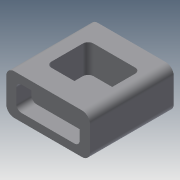
# Autodesk Inventor part: Part1
Saved by Autodesk Inventor 2015 (Build 190159000, 159)
## iProperties
Created: 2016-11-01
Part Number: Part1
Material: Generic
Document SubType Name: Modeling
Designer: Aniket Pant
Density: 1 g/cm^3
Appearance: Default
Author: Aniket Pant
Autodesk Inventor part; units mm, degrees
ref_plane "YZ Plane" through (0, 0, 0) normal (1, 0, 0) x (0, 1, 0)
ref_plane "XZ Plane" through (0, 0, 0) normal (0, 1, 0) x (-1, 0, 0)
ref_plane "XY Plane" through (0, 0, 0) normal (0, 0, 1) x (1, 0, 0)
sketch "Sketch1" plane through (0, 0, 0) normal (0, 0, 1) x (1, 0, 0)
  line L0 (7.62, 0) -> (72.898, 0)
  line L1 (80.518, 7.62) -> (80.518, 31.242)
  line L2 (72.898, 38.862) -> (7.62, 38.862)
  line L3 (0, 31.242) -> (0, 7.62)
  arc A0 (7.62, 38.862) -> (0, 31.242) centre (7.62, 31.242) ccw
  arc A1 (80.518, 31.242) -> (72.898, 38.862) centre (72.898, 31.242) ccw
  arc A2 (72.898, 0) -> (80.518, 7.62) centre (72.898, 7.62) ccw
  arc A3 (0, 7.62) -> (7.62, 0) centre (7.62, 7.62) ccw
  point P0 (0, 0)
  point P1 (80.518, 38.862)
  point P2 (80.518, 0)
  point P3 (0, 38.862)
  dimension "d0" = 80.518
  dimension "d1" = 38.862
  dimension "d2" = 7.62
  dimension "d3" = 7.62
  dimension "d4" = 7.62
  dimension "d5" = 7.62
  constraints: 8 end point, 8 point on circle, 8 point on line, 8 tangent, 4 centre point, 2 parallel, 1 horizontal, 1 perpendicular
  measures "d0" distance of point (80.518, 38.862) point (0, 38.862)
  measures "d1" distance of point (80.518, 0) point (80.518, 38.862)
  measures "d2" radius of A0
  measures "d3" radius of A1
  measures "d4" radius of A2
  measures "d5" radius of A3
extrude "Extrusion1" add sketch "Sketch1" along normal blind 80.518
sketch "Sketch2" plane through (7.62, 38.862, 0) normal (0, 1, 0) x (1, 0, 0)
  line L0 (14.986, -19.304) -> (55.118, -19.304)
  line L1 (60.198, -24.384) -> (60.198, -54.61)
  line L2 (55.118, -59.69) -> (14.986, -59.69)
  line L3 (9.906, -54.61) -> (9.906, -24.384)
  line L4 (65.278, -80.518) -> (0, -80.518) projected
  line L5 (72.898, 0) -> (72.898, -80.518) projected
  arc A0 (14.986, -19.304) -> (9.906, -24.384) centre (14.986, -24.384) ccw
  arc A1 (60.198, -24.384) -> (55.118, -19.304) centre (55.118, -24.384) ccw
  arc A2 (55.118, -59.69) -> (60.198, -54.61) centre (55.118, -54.61) ccw
  arc A3 (9.906, -54.61) -> (14.986, -59.69) centre (14.986, -54.61) ccw
  point P0 (-7.62, 0)
  point P1 (9.906, -19.304)
  point P2 (60.198, -19.304)
  point P3 (9.906, -59.69)
  dimension "d16" = 40.386
  dimension "d17" = 50.292
  dimension "d18" = 20.828
  dimension "d19" = 12.7
  dimension "d20" = 5.08
  dimension "d21" = 5.08
  dimension "d22" = 5.08
  dimension "d23" = 5.08
  constraints: 8 end point, 8 point on circle, 8 tangent, 6 point on line, 4 centre point, 2 parallel, 1 horizontal, 1 perpendicular
  measures "d16" distance of point (9.906, -59.69) point (9.906, -19.304)
  measures "d17" distance of point (9.906, -19.304) point (60.198, -19.304)
  measures "d18" distance between parallel lines of L4 L2
  measures "d19" distance between parallel lines of L5 L1
  measures "d20" radius of A0
  measures "d21" radius of A1
  measures "d22" radius of A2
  measures "d23" radius of A3
extrude "Extrusion2" cut sketch "Sketch2" against normal blind 27.178
sketch "Sketch3" plane through (0, 0, 80.518) normal (0, 0, 1) x (1, 0, 0)
  line L0 (14.732, 31.242) -> (65.532, 31.242)
  line L1 (70.612, 26.162) -> (70.612, 12.7)
  line L2 (65.532, 7.62) -> (14.732, 7.62)
  line L3 (9.652, 12.7) -> (9.652, 26.162)
  line L4 (80.518, 7.62) -> (80.518, 31.242) projected
  line L5 (72.898, 38.862) -> (7.62, 38.862) projected
  arc A0 (70.612, 26.162) -> (65.532, 31.242) centre (65.532, 26.162) ccw
  arc A1 (65.532, 7.62) -> (70.612, 12.7) centre (65.532, 12.7) ccw
  arc A2 (9.652, 12.7) -> (14.732, 7.62) centre (14.732, 12.7) ccw
  arc A3 (14.732, 31.242) -> (9.652, 26.162) centre (14.732, 26.162) ccw
  point P0 (0, 0)
  point P1 (9.652, 31.242)
  point P2 (70.612, 31.242)
  point P3 (9.652, 7.62)
  dimension "d26" = 60.96
  dimension "d27" = 9.906
  dimension "d28" = 23.622
  dimension "d29" = 7.62
  dimension "d30" = 5.08
  dimension "d31" = 5.08
  constraints: 8 end point, 8 point on circle, 8 tangent, 6 point on line, 4 centre point, 2 equal radius, 2 parallel, 1 horizontal, 1 perpendicular
  measures "d26" distance of point (9.652, 31.242) point (70.612, 31.242)
  measures "d27" distance between parallel lines of L4 L1
  measures "d28" distance of point (9.652, 7.62) point (9.652, 31.242)
  measures "d29" distance between parallel lines of L5 L0
  measures "d30" radius of A0
  measures "d31" radius of A1
extrude "Extrusion3" cut sketch "Sketch3" against normal blind 14.478
sketch "Sketch4" plane through (0, 0, 0) normal (0, 0, -1) x (-1, 0, 0)
  line L0 (-67.056, 32.004) -> (-13.716, 32.004)
  line L1 (-8.636, 26.924) -> (-8.636, 11.684)
  line L2 (-13.716, 6.604) -> (-67.056, 6.604)
  line L3 (-72.136, 11.684) -> (-72.136, 26.924)
  line L4 (0, 7.62) -> (0, 31.242) projected
  line L5 (-7.62, 38.862) -> (-72.898, 38.862) projected
  arc A0 (-67.056, 32.004) -> (-72.136, 26.924) centre (-67.056, 26.924) ccw
  arc A1 (-8.636, 26.924) -> (-13.716, 32.004) centre (-13.716, 26.924) ccw
  arc A2 (-13.716, 6.604) -> (-8.636, 11.684) centre (-13.716, 11.684) ccw
  arc A3 (-72.136, 11.684) -> (-67.056, 6.604) centre (-67.056, 11.684) ccw
  point P0 (0, 0)
  point P1 (-72.136, 32.004)
  point P2 (-8.636, 6.604)
  point P3 (-8.636, 32.004)
  dimension "d34" = 63.5
  dimension "d35" = 25.4
  dimension "d36" = 8.636
  dimension "d37" = 6.858
  dimension "d38" = 5.08
  constraints: 8 end point, 8 point on circle, 8 tangent, 6 point on line, 4 centre point, 3 equal radius, 2 parallel, 1 horizontal, 1 perpendicular
  measures "d34" distance of point (-72.136, 32.004) point (-8.636, 32.004)
  measures "d35" distance of point (-8.636, 32.004) point (-8.636, 6.604)
  measures "d36" distance between parallel lines of L4 L1
  measures "d37" distance between parallel lines of L5 L0
  measures "d38" radius of A0
extrude "Extrusion4" cut sketch "Sketch4" against normal blind 14.478
body "Solid1"
